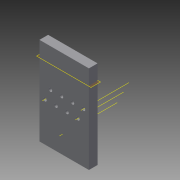
# Autodesk Inventor part: beep_rgb_ir
Saved by Autodesk Inventor 2014 (Build 180170000, 170)
## iProperties
Created: 2013-08-25
Part Number: beep_rgb_ir
Material: Generisch
Document SubType Name: Modeling
Designer: Felix
Density: 1 g/cm^3
Appearance: Vorgabe
Author: Felix
Autodesk Inventor part; units mm, degrees
ref_plane "YZ Plane" through (0, 0, 0) normal (1, 0, 0) x (0, 1, 0)
ref_plane "XZ Plane" through (0, 0, 0) normal (0, 1, 0) x (-1, 0, 0)
ref_plane "XY Plane" through (0, 0, 0) normal (0, 0, 1) x (1, 0, 0)
sketch "Skizze1" plane through (0, 0, 0) normal (0, 1, 0) x (-1, 0, 0)
  line L0 (0, 20.285) -> (0, 0)
  line L1 (11.4, 20.285) -> (0, 20.285)
  line L2 (11.4, 0) -> (11.4, 20.285)
  line L3 (0, 0) -> (11.4, 0)
  circle A0 centre (1.255, 11.57) radius 0.4064
  circle A1 centre (2.525, 9.03) radius 0.4064
  circle A2 centre (3.795, 11.57) radius 0.4064
  circle A3 centre (5.065, 9.03) radius 0.4064
  circle A4 centre (6.335, 11.57) radius 0.4064
  circle A5 centre (7.605, 9.03) radius 0.4064
  circle A6 centre (8.875, 11.57) radius 0.4064
  circle A7 centre (10.145, 9.03) radius 0.4064
  constraints: 8 centre point, 8 end point, 1 coincident
extrude "Extrusion1" add sketch "Skizze1" along normal blind 2
sketch "Skizze4" plane through (0, 2, 0) normal (0, 1, 0) x (1, 0, 0)
  circle A0 centre (-10.145, -9.03) radius 0.4064 projected
  circle A1 centre (-8.875, -11.57) radius 0.4064 projected
  circle A2 centre (-7.605, -9.03) radius 0.4064 projected
  circle A3 centre (-6.335, -11.57) radius 0.4064 projected
  circle A4 centre (-5.065, -9.03) radius 0.4064 projected
  circle A5 centre (-3.795, -11.57) radius 0.4064 projected
  circle A6 centre (-2.525, -9.03) radius 0.4064 projected
  circle A7 centre (-1.255, -11.57) radius 0.4064 projected
  line L0 (0, -20.285) -> (0, 0) projected
  line L1 (0, 0) -> (-11.4, 0) projected
  line L2 (-11.4, 0) -> (-11.4, -20.285) projected
  line L3 (-11.4, -20.285) -> (0, -20.285) projected
  line L4 (-11.4, -20.285) -> (-5.05, -20.285)
  line L5 (-5.05, -20.285) -> (-5.05, -16.8052)
  line L6 (-5.05, -16.8052) -> (-11.4, -16.8052)
  line L7 (-11.4, -16.8052) -> (-11.4, -20.285)
  line L8 (-11.4, -20.285) -> (-6.1, -20.285)
  line L9 (-6.1, -20.285) -> (-6.1, -4.085)
  line L10 (-6.1, -4.085) -> (-11.4, -4.085)
  line L11 (-11.4, -4.085) -> (-11.4, -20.285)
  dimension "d6" = 5.3
  dimension "d7" = 16.2
  dimension "d8" = 6.35
  dimension "d9" = 3.4798
  constraints: 16 end point, 4 parallel, 2 horizontal, 2 perpendicular
  measures "d6" distance of L9.end L10.end
  measures "d7" distance of L8.end L9.end
  measures "d8" distance of L5.end L6.end
  measures "d9" distance of L4.end L5.end
ref_plane "Arbeitsebene1" through (-5.05, 2, 16.8052) normal (0, 0, 1) x (1, 0, 0)
